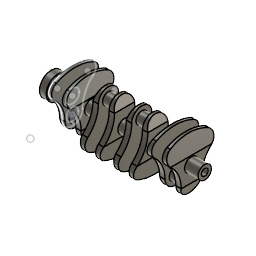
Arbore_cotit (Autodesk Fusion 360 design; units mm, degrees)
Autodesk Fusion 360 part; units mm, degrees
sketch "Sketch1" plane through (0, 0, 0) normal (1, 0, 0) x (0, 1, 0)
  circle A0 centre (0, 0) radius 17.5
  arc A1 (-30, 0) -> (-61.5875, 70.7379) centre (-125, 0) ccw
  arc A2 (56.125, 111.6915) -> (-56.125, 111.6915) centre (0, 0) ccw
  arc A3 (61.5875, 70.7379) -> (30, 0) centre (125, 0) ccw
  arc A4 (-56.125, 111.6915) -> (-61.5875, 70.7379) centre (-44.9, 89.3532) ccw
  arc A5 (61.5875, 70.7379) -> (56.125, 111.6915) centre (44.9, 89.3532) ccw
  arc A6 (-30, 0) -> (30, 0) centre (0, 0) ccw
  circle A7 centre (0, 47.5) radius 20
  dimension "d2" = 35
  dimension "d3" = 60
  dimension "d4" = 190
  dimension "d5" = 190
  dimension "d6" = 50
  dimension "d7" = 50
  dimension "d8" = 125
  dimension "d9" = 40
  dimension "d10" = 47.5
  constraint coincident A0.centre A2.centre
  constraint tangent A1 A4
  constraint tangent A3 A5
  constraint horizontal A0.centre A1.centre
  constraint horizontal A0.centre A3.centre
  constraint tangent A1 A6
  constraint tangent A3 A6
  constraint tangent A2 A4
  constraint tangent A2 A5
  constraint concentric A0 A6
  constraint concentric A2 A6
  constraint vertical A0.centre A7.centre
  measures "d2" diameter of A0
  measures "d3" diameter of A6
  measures "d4" diameter of A1
  measures "d5" diameter of A3
  measures "d6" diameter of A4
  measures "d7" diameter of A5
  measures "d8" radius of A2
  measures "d9" diameter of A7
  measures "d10" distance of A0.centre A7.centre
extrude "Extrude1" add sketch "Sketch1" along normal mid plane 16 contours A0 | A1 A2 A3 A4 A5 A6 | A7 makes body 1
extrude "Extrude2" add sketch "Sketch1" against normal blind 43 separate body contours A7 makes body 2
extrude "Extrude3" add sketch "Sketch1" along normal blind 40 separate body contours A0 makes body 3
extrude "Extrude4" add sketch "Sketch1" along normal blind 16 from surface at 40 separate body contours A0 | A1 A2 A3 A4 A5 A6 | A7 makes body 4
sketch "Sketch2" plane through (0, 0, 0) normal (0, 1, 0) x (1, 0, 0)
  line L0 (-8, 30) -> (-8, 0)
  line L1 (-8, 0) -> (-8, -70.7379)
  line L2 (-8, -70.7379) -> (-8, -111.6915)
  line L3 (-8, -111.6915) -> (-8, -125)
  line L4 (8, 0) -> (8, 30)
  line L5 (8, -70.7379) -> (8, 0)
  line L6 (8, -111.6915) -> (8, -70.7379)
  line L7 (8, -125) -> (8, -111.6915)
  line L8 (-8, 30) -> (8, 30)
  line L9 (-8, -125) -> (8, -125)
  line L10 (-43, -47.5) -> (-43, -67.5)
  line L11 (-43, -27.5) -> (-43, -47.5)
  line L12 (0, -47.5) -> (0, -27.5)
  line L13 (0, -67.5) -> (0, -47.5)
  line L14 (0, -27.5) -> (-43, -27.5)
  line L15 (0, -67.5) -> (-43, -67.5)
  line L16 (40, 0) -> (40, 17.5)
  line L17 (40, -17.5) -> (40, 0)
  line L18 (0, 0) -> (0, 17.5)
  line L19 (0, -17.5) -> (0, 0)
  line L20 (0, -17.5) -> (40, -17.5)
  line L21 (0, 17.5) -> (40, 17.5)
  line L22 (40, 0) -> (40, 30)
  line L23 (56, 0) -> (56, 30)
  line L24 (40, 0) -> (40, -70.7379)
  line L25 (56, -70.7379) -> (56, 0)
  line L26 (40, -111.6915) -> (40, -70.7379)
  line L27 (56, -111.6915) -> (56, -70.7379)
  line L28 (40, -125) -> (40, -111.6915)
  line L29 (56, -125) -> (56, -111.6915)
  line L30 (40, 30) -> (56, 30)
  line L31 (40, -125) -> (56, -125)
  line L32 (-8, -70.7379) -> (0, -125)
  line L33 (48, -125) -> (56, -70.7379)
  line L34 (48, 30) -> (56, 0)
  line L35 (0, 30) -> (-8, 0)
  constraint coincident L1.end L2.start
  constraint midpoint L9 L32.end
  constraint midpoint L31 L33.start
  constraint coincident L25.start L27.end
  constraint midpoint L30 L34.start
  constraint coincident L23.start L25.end
  constraint midpoint L8 L35.start
  constraint coincident L0.end L1.start
extrude "Extrude5" cut sketch "Sketch2" along normal through all and the other way through all contours L0 L8 L35 | L2 L3 L9 L32 | L23 L30 L34 | L27 L29 L31 L33 bodies 1 4
combine "Combine1" operation add target body 2 tool bodies 1 3 4
copy_body "CopyPasteBodies1" bodies 2 makes body 5
move_body "Move1" bodies 5 to x (1, 0, 0) y (0, -1, 0) z (0, 0, -1) at (99, 0, 95)
copy_body "CopyPasteBodies2" bodies 5 makes body 6
move_body "Move2" bodies 6 to x (1, 0, 0) y (0, 1, 0) z (0, 0, 1) at (99, 0, 0)
copy_body "CopyPasteBodies3" bodies 6 makes body 7
move_body "Move3" bodies 7 to x (1, 0, 0) y (0, -1, 0) z (0, 0, -1) at (99, 0, 95)
sketch "Sketch3" plane through (353, 0, 0) normal (1, 0, 0) x (0, 1, 0)
  line L0 (-30, 0) -> (30, 0)
  arc A0 (61.5875, 70.7379) -> (30, 0) centre (125, 0) ccw
  line L1 (61.5875, 70.7379) -> (-61.5875, 70.7379)
  arc A1 (-30, 0) -> (-61.5875, 70.7379) centre (-125, 0) ccw
  circle A2 centre (0, 47.5) radius 20
  circle A3 centre (0, 47.5) radius 10
  dimension "d22" = 40
  dimension "d23" = 20
  dimension "d24" = 47.5
  constraint concentric A2 A3
  constraint vertical A2.centre origin
  measures "d22" diameter of A2
  measures "d23" diameter of A3
  measures "d24" distance of A2.centre origin
extrude "Extrude6" add sketch "Sketch3" along normal blind 40 contours A2 bodies 7
sketch "Sketch4" plane through (-43, 0, 0) normal (-1, 0, 0) x (0, -1, 0)
  circle A0 centre (0, 47.5) radius 20
  circle A1 centre (0, 47.5) radius 35
  circle A2 centre (0, 75.5) radius 5
  circle A3 centre (-24.2487, 61.5) radius 5
  circle A4 centre (-24.2487, 33.5) radius 5
  circle A5 centre (0, 19.5) radius 5
  circle A6 centre (24.2487, 33.5) radius 5
  circle A7 centre (24.2487, 61.5) radius 5
  point P0 (0, 47.5)
  dimension "d27" = 70
  dimension "d28" = 10
  dimension "d29" = 28
  dimension "d31" = 360
  constraint concentric A0 A1
  constraint vertical A2.centre P0
  measures "d27" diameter of A1
  measures "d28" diameter of A2
  measures "d29" distance of P0 A2.centre
extrude "Extrude7" add sketch "Sketch4" along normal blind 20 contours A0 | A1 bodies 2
